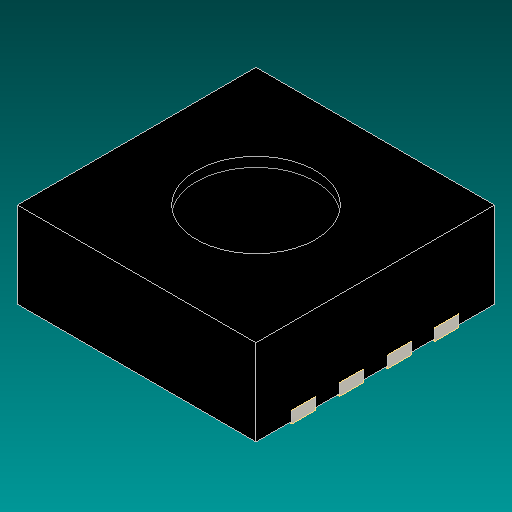
# Autodesk Inventor part: SHT3x-DIS
Saved by Autodesk Inventor 2017 (Build 210142000, 142)
## iProperties
Created: 2016-08-01
Part Number: SHT3x-DIS
Material: Generic
Document SubType Name: Modeling
Designer: Jonathan
Density: 1 g/cm^3
Appearance: Default
Author: Jonathan
Autodesk Inventor part; units mm, degrees
ref_plane "YZ Plane" through (0, 0, 0) normal (1, 0, 0) x (0, 1, 0)
ref_plane "XZ Plane" through (0, 0, 0) normal (0, 1, 0) x (-1, 0, 0)
ref_plane "XY Plane" through (0, 0, 0) normal (0, 0, 1) x (1, 0, 0)
sketch "Sketch1" plane through (0, 0, 0) normal (0, 1, 0) x (-1, 0, 0)
  line L0 (1.25, -1.25) -> (-1.25, -1.25)
  line L1 (-1.25, -1.25) -> (-1.25, 1.25)
  line L2 (-1.25, 1.25) -> (1.25, 1.25)
  line L3 (1.25, 1.25) -> (1.25, -1.25)
  line L4 (1.25, -1.25) -> (-1.25, 1.25) construction
  line L5 (-1.25, -1.25) -> (1.25, 1.25) construction
  point P0 (0, 0)
  dimension "d0" = 2.5
  constraints: 12 end point, 2 midpoint, 2 parallel, 2 perpendicular, 1 horizontal
  measures "d0" distance of L0.start L0.end
extrude "Extrusion1" add sketch "Sketch1" along normal blind 0.9
sketch "Sketch2" plane through (0, 0, 0) normal (0, -1, 0) x (1, 0, 0)
  line L0 (-1.25, -1.25) -> (-1.25, 1.25) projected
  line L1 (-1.25, 0.875) -> (-0.95, 0.875)
  line L2 (-1.25, 0.625) -> (-0.95, 0.625)
  arc A0 (-0.95, 0.625) -> (-0.95, 0.875) centre (-0.95, 0.75) ccw
  point P0 (0, 0)
  dimension "d3" = 0.25
  dimension "d4" = 0.3
  dimension "d6" = 0.875
  constraints: 4 end point, 2 horizontal, 2 point on circle, 2 point on line, 2 tangent, 1 centre point
  measures "d3" distance between parallel lines of L2 L1
  measures "d4" distance of L1.start L1.end
  measures "d6" distance from line of point (0, 0) L1
extrude "Extrusion2" cut sketch "Sketch2" against normal blind 0.1
pattern_linear "Rectangular Pattern1" count 4 spacing 0.5 along (0, 0, -1) of "Extrusion2"
extrude "Extrusion3" add sketch "Sketch2" against normal blind 0.1 and the other way blind 0.025 separate body
pattern_linear "Rectangular Pattern4" count 4 spacing 0.5 along (0, 0, -1) of "Extrusion3" bodies 2
mirror "Mirror1" about plane through (0, 0, 0) normal (1, 0, 0) of "Extrusion2", "Rectangular Pattern1" bodies 1
mirror "Mirror2" about plane through (0, 0, 0) normal (1, 0, 0) of "Extrusion3", "Rectangular Pattern4" bodies 2
sketch "Sketch3" plane through (0, 0, 0) normal (0, -1, 0) x (1, 0, 0)
  line L0 (-0.55, 0.9) -> (0.55, 0.9)
  line L1 (0.55, 0.9) -> (0.55, -0.9)
  line L2 (0.55, -0.9) -> (-0.55, -0.9)
  line L3 (-0.55, -0.9) -> (-0.55, 0.9)
  line L4 (-0.55, 0.9) -> (0.55, -0.9) construction
  line L5 (0.55, 0.9) -> (-0.55, -0.9) construction
  line L6 (0.3379, 0.9) -> (0.55, 0.6879)
  point P0 (0, 0)
  dimension "d23" = 45
  dimension "d24" = 0.3
  dimension "d25" = 1.8
  dimension "d26" = 1.1
  constraints: 14 end point, 2 midpoint, 2 parallel, 2 point on line, 1 horizontal, 1 perpendicular
  measures "d23" angle of L6 L0
  measures "d24" distance of L6.start L6.end
  measures "d25" distance of L0.end L1.end
  measures "d26" distance of L0.start L0.end
extrude "Extrusion4" cut sketch "Sketch3" against normal blind 0.1 contours L0 L6 L1 L2 L3 bodies 1
extrude "Extrusion5" add sketch "Sketch3" against normal blind 0.1 and the other way blind 0.025 contours L0 L6 L1 L2 L3 bodies 2
sketch "Sketch4" plane through (0, 0.9, 0) normal (0, 1, 0) x (1, 0, 0)
  circle A0 centre (0, 0) radius 0.625
  dimension "d31" = 1.25
  constraints: 1 centre point, 1 coincident
  measures "d31" diameter of A0
extrude "Extrusion6" cut sketch "Sketch4" against normal blind 0.1 bodies 1
body "Solid1"
body "Solid2"
